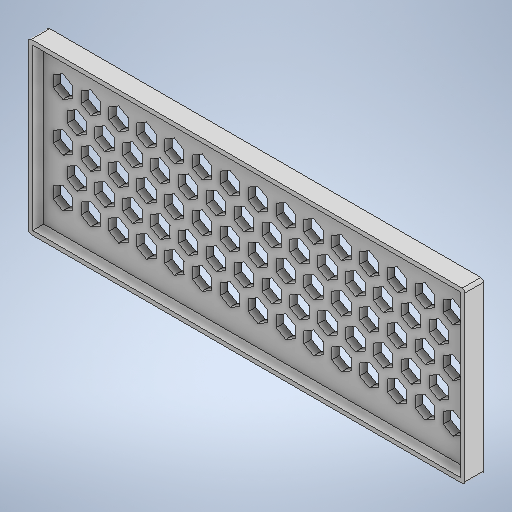
# Autodesk Inventor part: lm2596_box_lid_test
Saved by Autodesk Inventor 2025 (Build 290162000, 162)
## iProperties
Created: 2025-01-26
Part Number: lm2596_box_lid_test
Material: Všeobecné
Document SubType Name: Modeling
Designer: lukas
Density: 1 g/cm^3
Appearance: Výchozí
Author: lukas
## iProperties of the stored document lm2596_box_lid_3D tisk.ipt
Created: 2025-01-26
Part Number: lm2596_box_lid_3D tisk
Material: Všeobecné
Document SubType Name: Modeling
Designer: lukas
Density: 1 g/cm^3
Appearance: Výchozí
Author: lukas
Autodesk Inventor part; units mm, degrees
ref_plane "YZ Plane" through (0, 0, 0) normal (1, 0, 0) x (0, 1, 0)
ref_plane "XZ Plane" through (0, 0, 0) normal (0, 1, 0) x (-1, 0, 0)
ref_plane "XY Plane" through (0, 0, 0) normal (0, 0, 1) x (1, 0, 0)
sketch "Náčrt1" plane through (0, 0, 0) normal (0, 0, 1) x (1, 0, 0)
  line L0 (-117.5, 45.5) -> (117.5, 45.5)
  line L1 (117.5, 45.5) -> (117.5, -45.5)
  line L2 (117.5, -45.5) -> (-117.5, -45.5)
  line L3 (-117.5, -45.5) -> (-117.5, 45.5)
  line L4 (0, 63.7) -> (0, -63.7) projected
  line L5 (-164.5, 0) -> (164.5, 0) projected
  point P0 (0, 0)
  dimension "d0" = 235
  dimension "d1" = 91
  constraints: 8 end point, 2 parallel, 1 horizontal, 1 perpendicular, 2 other
  measures "d0" distance of L1.end L2.end
  measures "d1" distance of L0.end L1.end
extrude "Vysunutí1" add sketch "Náčrt1" along normal blind 4
sketch "Náčrt2" plane through (0, 0, 4) normal (0, 0, 1) x (1, 0, 0)
  line L0 (-117.5, 45.5) -> (-117.5, -45.5) projected
  line L1 (-117.5, -45.5) -> (117.5, -45.5) projected
  line L2 (117.5, -45.5) -> (117.5, 45.5) projected
  line L3 (117.5, 45.5) -> (-117.5, 45.5) projected
  line L4 (-164.5, 0) -> (164.5, 0) projected
  line L5 (0, -63.7) -> (0, 63.7) projected
  line L6 (-115.25, 43.25) -> (-115.25, -43.25)
  line L7 (-115.25, -43.25) -> (115.25, -43.25)
  line L8 (115.25, -43.25) -> (115.25, 43.25)
  line L9 (115.25, 43.25) -> (-115.25, 43.25)
  line L10 (-117.5, 45.5) -> (117.5, 45.5)
  line L11 (117.5, 45.5) -> (117.5, -45.5)
  line L12 (117.5, -45.5) -> (-117.5, -45.5)
  line L13 (-117.5, -45.5) -> (-117.5, 45.5)
  point P0 (0, 0)
  dimension "d5" = 2.25
  constraints: 16 end point, 2 parallel, 1 horizontal, 1 perpendicular, 3 other
  measures "d5" distance between parallel lines of L3 L9
extrude "Vysunutí2" add sketch "Náčrt2" along normal blind 6 contours L3 L5 L9 L6 L4 L0 | L4 L6 L7 L5 L1 L0 | L3 L2 L4 L8 L9 L5 | L5 L7 L8 L4 L2 L1
fillet "Zaoblení2" radius 1.5 4 edges at (117.5, -45.5, 5) (117.5, 45.5, 5) (-117.5, -45.5, 5) (-117.5, 45.5, 5)
sketch "Náčrt6" plane through (0, 0, 0) normal (0, 0, -1) x (-1, 0, 0)
  arc A0 (117.5, 44) -> (116, 45.5) centre (116, 44) ccw projected
  line L0 (-116, 45.5) -> (116, 45.5) projected
  arc A1 (-116, 45.5) -> (-117.5, 44) centre (-116, 44) ccw projected
  line L1 (-117.5, -44) -> (-117.5, 44) projected
  arc A2 (-117.5, -44) -> (-116, -45.5) centre (-116, -44) ccw projected
  line L2 (116, -45.5) -> (-116, -45.5) projected
  arc A3 (116, -45.5) -> (117.5, -44) centre (116, -44) ccw projected
  line L3 (117.5, 44) -> (117.5, -44) projected
  line L4 (0, -64.1349) -> (0, 64.1349) projected
  line L5 (-164.9349, 0) -> (164.9349, 0) projected
  line L6 (0, 6) -> (5.1962, 3)
  line L7 (5.1962, 3) -> (5.1962, -3)
  line L8 (5.1962, -3) -> (0, -6)
  line L9 (0, -6) -> (-5.1962, -3)
  line L10 (-5.1962, -3) -> (-5.1962, 3)
  line L11 (-5.1962, 3) -> (0, 6)
  line L12 (0, 0) -> (-2.5981, -4.5) construction
  line L13 (-7.5, -12.9904) -> (-10.0981, -17.4904) construction
  line L14 (-7.5, -18.9904) -> (-12.6962, -15.9904)
  line L15 (-12.6962, -15.9904) -> (-12.6962, -9.9904)
  line L16 (-2.3038, -9.9904) -> (-2.3038, -15.9904)
  line L17 (-12.6962, -9.9904) -> (-7.5, -6.9904)
  line L18 (-7.5, -6.9904) -> (-2.3038, -9.9904)
  line L19 (-2.3038, -15.9904) -> (-7.5, -18.9904)
  line L20 (-20.1962, 3) -> (-15, 6)
  line L21 (-15, 6) -> (-9.8038, 3)
  line L22 (-20.1962, -3) -> (-20.1962, 3)
  line L23 (-15, -6) -> (-20.1962, -3)
  line L24 (-9.8038, -3) -> (-15, -6)
  line L25 (-9.8038, 3) -> (-9.8038, -3)
  line L26 (9.8038, 3) -> (15, 6)
  line L27 (15, 6) -> (20.1962, 3)
  line L28 (9.8038, -3) -> (9.8038, 3)
  line L29 (15, -6) -> (9.8038, -3)
  line L30 (20.1962, -3) -> (15, -6)
  line L31 (20.1962, 3) -> (20.1962, -3)
  line L32 (-35.1962, 3) -> (-30, 6)
  line L33 (-30, 6) -> (-24.8038, 3)
  line L34 (-35.1962, -3) -> (-35.1962, 3)
  line L35 (-30, -6) -> (-35.1962, -3)
  line L36 (-24.8038, -3) -> (-30, -6)
  line L37 (-24.8038, 3) -> (-24.8038, -3)
  line L38 (24.8038, 3) -> (30, 6)
  line L39 (30, 6) -> (35.1962, 3)
  line L40 (24.8038, -3) -> (24.8038, 3)
  line L41 (30, -6) -> (24.8038, -3)
  line L42 (35.1962, -3) -> (30, -6)
  line L43 (35.1962, 3) -> (35.1962, -3)
  line L44 (-50.1962, 3) -> (-45, 6)
  line L45 (-45, 6) -> (-39.8038, 3)
  line L46 (-50.1962, -3) -> (-50.1962, 3)
  line L47 (-45, -6) -> (-50.1962, -3)
  line L48 (-39.8038, -3) -> (-45, -6)
  line L49 (-39.8038, 3) -> (-39.8038, -3)
  line L50 (39.8038, 3) -> (45, 6)
  line L51 (45, 6) -> (50.1962, 3)
  line L52 (39.8038, -3) -> (39.8038, 3)
  line L53 (45, -6) -> (39.8038, -3)
  line L54 (50.1962, -3) -> (45, -6)
  line L55 (50.1962, 3) -> (50.1962, -3)
  line L56 (-65.1962, 3) -> (-60, 6)
  line L57 (-60, 6) -> (-54.8038, 3)
  line L58 (-65.1962, -3) -> (-65.1962, 3)
  line L59 (-60, -6) -> (-65.1962, -3)
  line L60 (-54.8038, -3) -> (-60, -6)
  line L61 (-54.8038, 3) -> (-54.8038, -3)
  line L62 (54.8038, 3) -> (60, 6)
  line L63 (60, 6) -> (65.1962, 3)
  line L64 (54.8038, -3) -> (54.8038, 3)
  line L65 (60, -6) -> (54.8038, -3)
  line L66 (65.1962, -3) -> (60, -6)
  line L67 (65.1962, 3) -> (65.1962, -3)
  line L68 (-80.1962, 3) -> (-75, 6)
  line L69 (-75, 6) -> (-69.8038, 3)
  line L70 (-80.1962, -3) -> (-80.1962, 3)
  line L71 (-75, -6) -> (-80.1962, -3)
  line L72 (-69.8038, -3) -> (-75, -6)
  line L73 (-69.8038, 3) -> (-69.8038, -3)
  line L74 (69.8038, 3) -> (75, 6)
  line L75 (75, 6) -> (80.1962, 3)
  line L76 (69.8038, -3) -> (69.8038, 3)
  line L77 (75, -6) -> (69.8038, -3)
  line L78 (80.1962, -3) -> (75, -6)
  line L79 (80.1962, 3) -> (80.1962, -3)
  line L80 (-95.1962, 3) -> (-90, 6)
  line L81 (-90, 6) -> (-84.8038, 3)
  line L82 (-95.1962, -3) -> (-95.1962, 3)
  line L83 (-90, -6) -> (-95.1962, -3)
  line L84 (-84.8038, -3) -> (-90, -6)
  line L85 (-84.8038, 3) -> (-84.8038, -3)
  line L86 (84.8038, 3) -> (90, 6)
  line L87 (90, 6) -> (95.1962, 3)
  line L88 (84.8038, -3) -> (84.8038, 3)
  line L89 (90, -6) -> (84.8038, -3)
  line L90 (95.1962, -3) -> (90, -6)
  line L91 (95.1962, 3) -> (95.1962, -3)
  line L92 (-110.1962, 3) -> (-105, 6)
  line L93 (-105, 6) -> (-99.8038, 3)
  line L94 (-110.1962, -3) -> (-110.1962, 3)
  line L95 (-105, -6) -> (-110.1962, -3)
  line L96 (-99.8038, -3) -> (-105, -6)
  line L97 (-99.8038, 3) -> (-99.8038, -3)
  line L98 (99.8038, 3) -> (105, 6)
  line L99 (105, 6) -> (110.1962, 3)
  line L100 (99.8038, -3) -> (99.8038, 3)
  line L101 (105, -6) -> (99.8038, -3)
  line L102 (110.1962, -3) -> (105, -6)
  line L103 (110.1962, 3) -> (110.1962, -3)
  line L104 (7.5, -12.9904) -> (4.9019, -17.4904) construction
  line L105 (2.3038, -9.9904) -> (7.5, -6.9904)
  line L106 (2.3038, -15.9904) -> (2.3038, -9.9904)
  line L107 (7.5, -18.9904) -> (2.3038, -15.9904)
  line L108 (12.6962, -15.9904) -> (7.5, -18.9904)
  line L109 (7.5, -6.9904) -> (12.6962, -9.9904)
  line L110 (12.6962, -9.9904) -> (12.6962, -15.9904)
  line L111 (22.5, -12.9904) -> (19.9019, -17.4904) construction
  line L112 (17.3038, -9.9904) -> (22.5, -6.9904)
  line L113 (17.3038, -15.9904) -> (17.3038, -9.9904)
  line L114 (22.5, -18.9904) -> (17.3038, -15.9904)
  line L115 (27.6962, -15.9904) -> (22.5, -18.9904)
  line L116 (22.5, -6.9904) -> (27.6962, -9.9904)
  line L117 (27.6962, -9.9904) -> (27.6962, -15.9904)
  line L118 (37.5, -12.9904) -> (34.9019, -17.4904) construction
  line L119 (32.3038, -9.9904) -> (37.5, -6.9904)
  line L120 (32.3038, -15.9904) -> (32.3038, -9.9904)
  line L121 (37.5, -18.9904) -> (32.3038, -15.9904)
  line L122 (42.6962, -15.9904) -> (37.5, -18.9904)
  line L123 (37.5, -6.9904) -> (42.6962, -9.9904)
  line L124 (42.6962, -9.9904) -> (42.6962, -15.9904)
  line L125 (52.5, -12.9904) -> (49.9019, -17.4904) construction
  line L126 (47.3038, -9.9904) -> (52.5, -6.9904)
  line L127 (47.3038, -15.9904) -> (47.3038, -9.9904)
  line L128 (52.5, -18.9904) -> (47.3038, -15.9904)
  line L129 (57.6962, -15.9904) -> (52.5, -18.9904)
  line L130 (52.5, -6.9904) -> (57.6962, -9.9904)
  line L131 (57.6962, -9.9904) -> (57.6962, -15.9904)
  line L132 (67.5, -12.9904) -> (64.9019, -17.4904) construction
  line L133 (62.3038, -9.9904) -> (67.5, -6.9904)
  line L134 (62.3038, -15.9904) -> (62.3038, -9.9904)
  line L135 (67.5, -18.9904) -> (62.3038, -15.9904)
  line L136 (72.6962, -15.9904) -> (67.5, -18.9904)
  line L137 (67.5, -6.9904) -> (72.6962, -9.9904)
  line L138 (72.6962, -9.9904) -> (72.6962, -15.9904)
  line L139 (82.5, -12.9904) -> (79.9019, -17.4904) construction
  line L140 (77.3038, -9.9904) -> (82.5, -6.9904)
  line L141 (77.3038, -15.9904) -> (77.3038, -9.9904)
  line L142 (82.5, -18.9904) -> (77.3038, -15.9904)
  line L143 (87.6962, -15.9904) -> (82.5, -18.9904)
  line L144 (82.5, -6.9904) -> (87.6962, -9.9904)
  line L145 (87.6962, -9.9904) -> (87.6962, -15.9904)
  line L146 (97.5, -12.9904) -> (94.9019, -17.4904) construction
  line L147 (92.3038, -9.9904) -> (97.5, -6.9904)
  line L148 (92.3038, -15.9904) -> (92.3038, -9.9904)
  line L149 (97.5, -18.9904) -> (92.3038, -15.9904)
  line L150 (102.6962, -15.9904) -> (97.5, -18.9904)
  line L151 (97.5, -6.9904) -> (102.6962, -9.9904)
  line L152 (102.6962, -9.9904) -> (102.6962, -15.9904)
  line L153 (-27.6962, -9.9904) -> (-22.5, -6.9904)
  line L154 (-22.5, -6.9904) -> (-17.3038, -9.9904)
  line L155 (-27.6962, -15.9904) -> (-27.6962, -9.9904)
  line L156 (-22.5, -12.9904) -> (-25.0981, -17.4904) construction
  line L157 (-22.5, -18.9904) -> (-27.6962, -15.9904)
  line L158 (-17.3038, -15.9904) -> (-22.5, -18.9904)
  line L159 (-17.3038, -9.9904) -> (-17.3038, -15.9904)
  line L160 (-42.6962, -9.9904) -> (-37.5, -6.9904)
  line L161 (-37.5, -6.9904) -> (-32.3038, -9.9904)
  line L162 (-42.6962, -15.9904) -> (-42.6962, -9.9904)
  line L163 (-37.5, -12.9904) -> (-40.0981, -17.4904) construction
  line L164 (-37.5, -18.9904) -> (-42.6962, -15.9904)
  line L165 (-32.3038, -15.9904) -> (-37.5, -18.9904)
  line L166 (-32.3038, -9.9904) -> (-32.3038, -15.9904)
  line L167 (-57.6962, -9.9904) -> (-52.5, -6.9904)
  line L168 (-52.5, -6.9904) -> (-47.3038, -9.9904)
  line L169 (-57.6962, -15.9904) -> (-57.6962, -9.9904)
  line L170 (-52.5, -12.9904) -> (-55.0981, -17.4904) construction
  line L171 (-52.5, -18.9904) -> (-57.6962, -15.9904)
  line L172 (-47.3038, -15.9904) -> (-52.5, -18.9904)
  line L173 (-47.3038, -9.9904) -> (-47.3038, -15.9904)
  line L174 (-72.6962, -9.9904) -> (-67.5, -6.9904)
  line L175 (-67.5, -6.9904) -> (-62.3038, -9.9904)
  line L176 (-72.6962, -15.9904) -> (-72.6962, -9.9904)
  line L177 (-67.5, -12.9904) -> (-70.0981, -17.4904) construction
  line L178 (-67.5, -18.9904) -> (-72.6962, -15.9904)
  line L179 (-62.3038, -15.9904) -> (-67.5, -18.9904)
  line L180 (-62.3038, -9.9904) -> (-62.3038, -15.9904)
  line L181 (-87.6962, -9.9904) -> (-82.5, -6.9904)
  line L182 (-82.5, -6.9904) -> (-77.3038, -9.9904)
  line L183 (-87.6962, -15.9904) -> (-87.6962, -9.9904)
  line L184 (-82.5, -12.9904) -> (-85.0981, -17.4904) construction
  line L185 (-82.5, -18.9904) -> (-87.6962, -15.9904)
  line L186 (-77.3038, -15.9904) -> (-82.5, -18.9904)
  line L187 (-77.3038, -9.9904) -> (-77.3038, -15.9904)
  line L188 (-102.6962, -9.9904) -> (-97.5, -6.9904)
  line L189 (-97.5, -6.9904) -> (-92.3038, -9.9904)
  line L190 (-102.6962, -15.9904) -> (-102.6962, -9.9904)
  line L191 (-97.5, -12.9904) -> (-100.0981, -17.4904) construction
  line L192 (-97.5, -18.9904) -> (-102.6962, -15.9904)
  line L193 (-92.3038, -15.9904) -> (-97.5, -18.9904)
  line L194 (-92.3038, -9.9904) -> (-92.3038, -15.9904)
  line L195 (-12.6962, 15.9896) -> (-7.5, 18.9896)
  line L196 (-7.5, 18.9896) -> (-2.3038, 15.9896)
  line L197 (-2.3038, 15.9896) -> (-2.3038, 9.9896)
  line L198 (-2.3038, 9.9896) -> (-7.5, 6.9896)
  line L199 (-7.5, 12.9896) -> (-10.0981, 8.4896) construction
  line L200 (-7.5, 6.9896) -> (-12.6962, 9.9896)
  line L201 (-12.6962, 9.9896) -> (-12.6962, 15.9896)
  line L202 (2.3038, 9.9896) -> (2.3038, 15.9896)
  line L203 (7.5, 6.9896) -> (2.3038, 9.9896)
  line L204 (2.3038, 15.9896) -> (7.5, 18.9896)
  line L205 (7.5, 12.9896) -> (4.9019, 8.4896) construction
  line L206 (12.6962, 9.9896) -> (7.5, 6.9896)
  line L207 (12.6962, 15.9896) -> (12.6962, 9.9896)
  line L208 (7.5, 18.9896) -> (12.6962, 15.9896)
  line L209 (32.3038, 15.9896) -> (37.5, 18.9896)
  line L210 (37.5, 18.9896) -> (42.6962, 15.9896)
  line L211 (32.3038, 9.9896) -> (32.3038, 15.9896)
  line L212 (42.6962, 15.9896) -> (42.6962, 9.9896)
  line L213 (37.5, 12.9896) -> (34.9019, 8.4896) construction
  line L214 (37.5, 6.9896) -> (32.3038, 9.9896)
  line L215 (42.6962, 9.9896) -> (37.5, 6.9896)
  line L216 (-42.6962, 15.9896) -> (-37.5, 18.9896)
  line L217 (-37.5, 18.9896) -> (-32.3038, 15.9896)
  line L218 (-32.3038, 15.9896) -> (-32.3038, 9.9896)
  line L219 (-32.3038, 9.9896) -> (-37.5, 6.9896)
  line L220 (-37.5, 12.9896) -> (-40.0981, 8.4896) construction
  line L221 (-42.6962, 9.9896) -> (-42.6962, 15.9896)
  line L222 (-37.5, 6.9896) -> (-42.6962, 9.9896)
  line L223 (62.3038, 15.9896) -> (67.5, 18.9896)
  line L224 (62.3038, 9.9896) -> (62.3038, 15.9896)
  line L225 (67.5, 18.9896) -> (72.6962, 15.9896)
  line L226 (67.5, 6.9896) -> (62.3038, 9.9896)
  line L227 (72.6962, 15.9896) -> (72.6962, 9.9896)
  line L228 (72.6962, 9.9896) -> (67.5, 6.9896)
  line L229 (67.5, 12.9896) -> (64.9019, 8.4896) construction
  line L230 (-67.5, 18.9896) -> (-62.3038, 15.9896)
  line L231 (-57.6962, 15.9896) -> (-52.5, 18.9896)
  line L232 (-62.3038, 15.9896) -> (-62.3038, 9.9896)
  line L233 (-62.3038, 9.9896) -> (-67.5, 6.9896)
  line L234 (-52.5, 18.9896) -> (-47.3038, 15.9896)
  line L235 (-57.6962, 9.9896) -> (-57.6962, 15.9896)
  line L236 (-52.5, 12.9896) -> (-55.0981, 8.4896) construction
  line L237 (-47.3038, 15.9896) -> (-47.3038, 9.9896)
  line L238 (-47.3038, 9.9896) -> (-52.5, 6.9896)
  line L239 (-52.5, 6.9896) -> (-57.6962, 9.9896)
  line L240 (-82.5, 12.9896) -> (-85.0981, 8.4896) construction
  line L241 (-82.5, 6.9896) -> (-87.6962, 9.9896)
  line L242 (-87.6962, 15.9896) -> (-82.5, 18.9896)
  line L243 (-87.6962, 9.9896) -> (-87.6962, 15.9896)
  line L244 (92.3038, 15.9896) -> (97.5, 18.9896)
  line L245 (87.6962, 15.9896) -> (87.6962, 9.9896)
  line L246 (92.3038, 9.9896) -> (92.3038, 15.9896)
  line L247 (97.5, 18.9896) -> (102.6962, 15.9896)
  line L248 (97.5, 12.9896) -> (94.9019, 8.4896) construction
  line L249 (97.5, 6.9896) -> (92.3038, 9.9896)
  line L250 (102.6962, 15.9896) -> (102.6962, 9.9896)
  line L251 (102.6962, 9.9896) -> (97.5, 6.9896)
  line L252 (77.3038, 9.9896) -> (77.3038, 15.9896)
  line L253 (82.5, 6.9896) -> (77.3038, 9.9896)
  line L254 (82.5, 12.9896) -> (79.9019, 8.4896) construction
  line L255 (77.3038, 15.9896) -> (82.5, 18.9896)
  line L256 (82.5, 18.9896) -> (87.6962, 15.9896)
  line L257 (87.6962, 9.9896) -> (82.5, 6.9896)
  line L258 (-102.6962, 15.9896) -> (-97.5, 18.9896)
  line L259 (-97.5, 18.9896) -> (-92.3038, 15.9896)
  line L260 (-102.6962, 9.9896) -> (-102.6962, 15.9896)
  line L261 (-97.5, 12.9896) -> (-100.0981, 8.4896) construction
  line L262 (-97.5, 6.9896) -> (-102.6962, 9.9896)
  line L263 (-92.3038, 15.9896) -> (-92.3038, 9.9896)
  line L264 (-92.3038, 9.9896) -> (-97.5, 6.9896)
  line L265 (47.3038, 9.9896) -> (47.3038, 15.9896)
  line L266 (47.3038, 15.9896) -> (52.5, 18.9896)
  line L267 (52.5, 6.9896) -> (47.3038, 9.9896)
  line L268 (52.5, 12.9896) -> (49.9019, 8.4896) construction
  line L269 (52.5, 18.9896) -> (57.6962, 15.9896)
  line L270 (57.6962, 15.9896) -> (57.6962, 9.9896)
  line L271 (57.6962, 9.9896) -> (52.5, 6.9896)
  line L272 (-27.6962, 9.9896) -> (-27.6962, 15.9896)
  line L273 (-27.6962, 15.9896) -> (-22.5, 18.9896)
  line L274 (-22.5, 18.9896) -> (-17.3038, 15.9896)
  line L275 (-22.5, 12.9896) -> (-25.0981, 8.4896) construction
  line L276 (-22.5, 6.9896) -> (-27.6962, 9.9896)
  line L277 (-17.3038, 15.9896) -> (-17.3038, 9.9896)
  line L278 (-17.3038, 9.9896) -> (-22.5, 6.9896)
  line L279 (-77.3038, 9.9896) -> (-82.5, 6.9896)
  line L280 (-82.5, 18.9896) -> (-77.3038, 15.9896)
  line L281 (-77.3038, 15.9896) -> (-77.3038, 9.9896)
  line L282 (-72.6962, 9.9896) -> (-72.6962, 15.9896)
  line L283 (-72.6962, 15.9896) -> (-67.5, 18.9896)
  line L284 (-67.5, 12.9896) -> (-70.0981, 8.4896) construction
  line L285 (-67.5, 6.9896) -> (-72.6962, 9.9896)
  line L286 (17.3038, 9.9896) -> (17.3038, 15.9896)
  line L287 (22.5, 6.9896) -> (17.3038, 9.9896)
  line L288 (17.3038, 15.9896) -> (22.5, 18.9896)
  line L289 (22.5, 12.9896) -> (19.9019, 8.4896) construction
  line L290 (27.6962, 15.9896) -> (27.6962, 9.9896)
  line L291 (22.5, 18.9896) -> (27.6962, 15.9896)
  line L292 (27.6962, 9.9896) -> (22.5, 6.9896)
  line L293 (84.8038, 28.98) -> (90, 31.98)
  line L294 (75, 31.98) -> (80.1962, 28.98)
  line L295 (-50.1962, 22.98) -> (-50.1962, 28.98)
  line L296 (-65.1962, 28.98) -> (-60, 31.98)
  line L297 (-60, 31.98) -> (-54.8038, 28.98)
  line L298 (-60, 19.98) -> (-65.1962, 22.98)
  line L299 (-54.8038, 22.98) -> (-60, 19.98)
  line L300 (-54.8038, 28.98) -> (-54.8038, 22.98)
  line L301 (-69.8038, 28.98) -> (-69.8038, 22.98)
  line L302 (-75, 31.98) -> (-69.8038, 28.98)
  line L303 (-45, 19.98) -> (-50.1962, 22.98)
  line L304 (-39.8038, 22.98) -> (-45, 19.98)
  line L305 (-35.1962, 28.98) -> (-30, 31.98)
  line L306 (-30, 31.98) -> (-24.8038, 28.98)
  line L307 (-35.1962, 22.98) -> (-35.1962, 28.98)
  line L308 (-39.8038, 28.98) -> (-39.8038, 22.98)
  line L309 (-24.8038, 28.98) -> (-24.8038, 22.98)
  line L310 (-30, 19.98) -> (-35.1962, 22.98)
  line L311 (-24.8038, 22.98) -> (-30, 19.98)
  line L312 (-5.1962, 22.98) -> (-5.1962, 28.98)
  line L313 (-20.1962, 28.98) -> (-15, 31.98)
  line L314 (-15, 31.98) -> (-9.8038, 28.98)
  line L315 (-20.1962, 22.98) -> (-20.1962, 28.98)
  line L316 (-15, 19.98) -> (-20.1962, 22.98)
  line L317 (-9.8038, 28.98) -> (-9.8038, 22.98)
  line L318 (-9.8038, 22.98) -> (-15, 19.98)
  line L319 (-5.1962, 28.98) -> (0, 31.98)
  line L320 (0, 25.98) -> (-2.5981, 21.48) construction
  line L321 (5.1962, 28.98) -> (5.1962, 22.98)
  line L322 (0, 31.98) -> (5.1962, 28.98)
  line L323 (5.1962, 22.98) -> (0, 19.98)
  line L324 (0, 19.98) -> (-5.1962, 22.98)
  line L325 (15, 19.98) -> (9.8038, 22.98)
  line L326 (9.8038, 28.98) -> (15, 31.98)
  line L327 (15, 31.98) -> (20.1962, 28.98)
  line L328 (9.8038, 22.98) -> (9.8038, 28.98)
  line L329 (20.1962, 22.98) -> (15, 19.98)
  line L330 (20.1962, 28.98) -> (20.1962, 22.98)
  line L331 (24.8038, 28.98) -> (30, 31.98)
  line L332 (24.8038, 22.98) -> (24.8038, 28.98)
  line L333 (30, 19.98) -> (24.8038, 22.98)
  line L334 (30, 31.98) -> (35.1962, 28.98)
  line L335 (35.1962, 22.98) -> (30, 19.98)
  line L336 (45, 19.98) -> (39.8038, 22.98)
  line L337 (50.1962, 22.98) -> (45, 19.98)
  line L338 (50.1962, 28.98) -> (50.1962, 22.98)
  line L339 (45, 31.98) -> (50.1962, 28.98)
  line L340 (39.8038, 22.98) -> (39.8038, 28.98)
  line L341 (35.1962, 28.98) -> (35.1962, 22.98)
  line L342 (39.8038, 28.98) -> (45, 31.98)
  line L343 (54.8038, 22.98) -> (54.8038, 28.98)
  line L344 (60, 19.98) -> (54.8038, 22.98)
  line L345 (54.8038, 28.98) -> (60, 31.98)
  line L346 (60, 31.98) -> (65.1962, 28.98)
  line L347 (65.1962, 22.98) -> (60, 19.98)
  line L348 (75, 19.98) -> (69.8038, 22.98)
  line L349 (80.1962, 22.98) -> (75, 19.98)
  line L350 (69.8038, 22.98) -> (69.8038, 28.98)
  line L351 (65.1962, 28.98) -> (65.1962, 22.98)
  line L352 (69.8038, 28.98) -> (75, 31.98)
  line L353 (80.1962, 28.98) -> (80.1962, 22.98)
  line L354 (84.8038, 22.98) -> (84.8038, 28.98)
  line L355 (90, 19.98) -> (84.8038, 22.98)
  line L356 (105, 19.98) -> (99.8038, 22.98)
  line L357 (95.1962, 22.98) -> (90, 19.98)
  line L358 (95.1962, 28.98) -> (95.1962, 22.98)
  line L359 (90, 31.98) -> (95.1962, 28.98)
  line L360 (110.1962, 22.98) -> (105, 19.98)
  line L361 (99.8038, 22.98) -> (99.8038, 28.98)
  line L362 (110.1962, 28.98) -> (110.1962, 22.98)
  line L363 (99.8038, 28.98) -> (105, 31.98)
  line L364 (105, 31.98) -> (110.1962, 28.98)
  line L365 (-45, 31.98) -> (-39.8038, 28.98)
  line L366 (-50.1962, 28.98) -> (-45, 31.98)
  line L367 (-95.1962, 28.98) -> (-90, 31.98)
  line L368 (-90, 31.98) -> (-84.8038, 28.98)
  line L369 (-95.1962, 22.98) -> (-95.1962, 28.98)
  line L370 (-90, 19.98) -> (-95.1962, 22.98)
  line L371 (-105, 31.98) -> (-99.8038, 28.98)
  line L372 (-84.8038, 28.98) -> (-84.8038, 22.98)
  line L373 (-84.8038, 22.98) -> (-90, 19.98)
  line L374 (-110.1962, 28.98) -> (-105, 31.98)
  line L375 (-99.8038, 28.98) -> (-99.8038, 22.98)
  line L376 (-99.8038, 22.98) -> (-105, 19.98)
  line L377 (-110.1962, 22.98) -> (-110.1962, 28.98)
  line L378 (-105, 19.98) -> (-110.1962, 22.98)
  line L379 (-75, 19.98) -> (-80.1962, 22.98)
  line L380 (-80.1962, 22.98) -> (-80.1962, 28.98)
  line L381 (-80.1962, 28.98) -> (-75, 31.98)
  line L382 (-65.1962, 22.98) -> (-65.1962, 28.98)
  line L383 (-69.8038, 22.98) -> (-75, 19.98)
  line L384 (84.8038, -22.98) -> (90, -19.98)
  line L385 (75, -19.98) -> (80.1962, -22.98)
  line L386 (-50.1962, -28.98) -> (-50.1962, -22.98)
  line L387 (-65.1962, -22.98) -> (-60, -19.98)
  line L388 (-60, -19.98) -> (-54.8038, -22.98)
  line L389 (-60, -31.98) -> (-65.1962, -28.98)
  line L390 (-54.8038, -28.98) -> (-60, -31.98)
  line L391 (-54.8038, -22.98) -> (-54.8038, -28.98)
  line L392 (-69.8038, -22.98) -> (-69.8038, -28.98)
  line L393 (-75, -19.98) -> (-69.8038, -22.98)
  line L394 (-45, -31.98) -> (-50.1962, -28.98)
  line L395 (-39.8038, -28.98) -> (-45, -31.98)
  line L396 (-35.1962, -22.98) -> (-30, -19.98)
  line L397 (-30, -19.98) -> (-24.8038, -22.98)
  line L398 (-35.1962, -28.98) -> (-35.1962, -22.98)
  line L399 (-39.8038, -22.98) -> (-39.8038, -28.98)
  line L400 (-24.8038, -22.98) -> (-24.8038, -28.98)
  line L401 (-30, -31.98) -> (-35.1962, -28.98)
  line L402 (-24.8038, -28.98) -> (-30, -31.98)
  line L403 (-5.1962, -28.98) -> (-5.1962, -22.98)
  line L404 (-20.1962, -22.98) -> (-15, -19.98)
  line L405 (-15, -19.98) -> (-9.8038, -22.98)
  line L406 (-20.1962, -28.98) -> (-20.1962, -22.98)
  line L407 (-15, -31.98) -> (-20.1962, -28.98)
  line L408 (-9.8038, -22.98) -> (-9.8038, -28.98)
  line L409 (-9.8038, -28.98) -> (-15, -31.98)
  line L410 (-5.1962, -22.98) -> (0, -19.98)
  line L411 (0, -25.98) -> (-2.5981, -30.48) construction
  line L412 (5.1962, -22.98) -> (5.1962, -28.98)
  line L413 (0, -19.98) -> (5.1962, -22.98)
  line L414 (5.1962, -28.98) -> (0, -31.98)
  line L415 (0, -31.98) -> (-5.1962, -28.98)
  line L416 (15, -31.98) -> (9.8038, -28.98)
  line L417 (9.8038, -22.98) -> (15, -19.98)
  line L418 (15, -19.98) -> (20.1962, -22.98)
  line L419 (9.8038, -28.98) -> (9.8038, -22.98)
  line L420 (20.1962, -28.98) -> (15, -31.98)
  line L421 (20.1962, -22.98) -> (20.1962, -28.98)
  line L422 (24.8038, -22.98) -> (30, -19.98)
  line L423 (24.8038, -28.98) -> (24.8038, -22.98)
  line L424 (30, -31.98) -> (24.8038, -28.98)
  line L425 (30, -19.98) -> (35.1962, -22.98)
  line L426 (35.1962, -28.98) -> (30, -31.98)
  line L427 (45, -31.98) -> (39.8038, -28.98)
  line L428 (50.1962, -28.98) -> (45, -31.98)
  line L429 (50.1962, -22.98) -> (50.1962, -28.98)
  line L430 (45, -19.98) -> (50.1962, -22.98)
  line L431 (39.8038, -28.98) -> (39.8038, -22.98)
  line L432 (35.1962, -22.98) -> (35.1962, -28.98)
  line L433 (39.8038, -22.98) -> (45, -19.98)
  line L434 (54.8038, -28.98) -> (54.8038, -22.98)
  line L435 (60, -31.98) -> (54.8038, -28.98)
  line L436 (54.8038, -22.98) -> (60, -19.98)
  line L437 (60, -19.98) -> (65.1962, -22.98)
  line L438 (65.1962, -28.98) -> (60, -31.98)
  line L439 (75, -31.98) -> (69.8038, -28.98)
  line L440 (80.1962, -28.98) -> (75, -31.98)
  line L441 (69.8038, -28.98) -> (69.8038, -22.98)
  line L442 (65.1962, -22.98) -> (65.1962, -28.98)
  line L443 (69.8038, -22.98) -> (75, -19.98)
  line L444 (80.1962, -22.98) -> (80.1962, -28.98)
  line L445 (84.8038, -28.98) -> (84.8038, -22.98)
  line L446 (90, -31.98) -> (84.8038, -28.98)
  line L447 (105, -31.98) -> (99.8038, -28.98)
  line L448 (95.1962, -28.98) -> (90, -31.98)
  line L449 (95.1962, -22.98) -> (95.1962, -28.98)
  line L450 (90, -19.98) -> (95.1962, -22.98)
  line L451 (110.1962, -28.98) -> (105, -31.98)
  line L452 (99.8038, -28.98) -> (99.8038, -22.98)
  line L453 (110.1962, -22.98) -> (110.1962, -28.98)
  line L454 (99.8038, -22.98) -> (105, -19.98)
  line L455 (105, -19.98) -> (110.1962, -22.98)
  line L456 (-45, -19.98) -> (-39.8038, -22.98)
  line L457 (-50.1962, -22.98) -> (-45, -19.98)
  line L458 (-95.1962, -22.98) -> (-90, -19.98)
  line L459 (-90, -19.98) -> (-84.8038, -22.98)
  line L460 (-95.1962, -28.98) -> (-95.1962, -22.98)
  line L461 (-90, -31.98) -> (-95.1962, -28.98)
  line L462 (-105, -19.98) -> (-99.8038, -22.98)
  line L463 (-84.8038, -22.98) -> (-84.8038, -28.98)
  line L464 (-84.8038, -28.98) -> (-90, -31.98)
  line L465 (-110.1962, -22.98) -> (-105, -19.98)
  line L466 (-99.8038, -22.98) -> (-99.8038, -28.98)
  line L467 (-99.8038, -28.98) -> (-105, -31.98)
  line L468 (-110.1962, -28.98) -> (-110.1962, -22.98)
  line L469 (-105, -31.98) -> (-110.1962, -28.98)
  line L470 (-75, -31.98) -> (-80.1962, -28.98)
  line L471 (-80.1962, -28.98) -> (-80.1962, -22.98)
  line L472 (-80.1962, -22.98) -> (-75, -19.98)
  line L473 (-65.1962, -28.98) -> (-65.1962, -22.98)
  line L474 (-69.8038, -28.98) -> (-75, -31.98)
  point P0 (-15, 0)
  point P1 (-17.5981, -4.5)
  point P2 (15, 0)
  point P3 (12.4019, -4.5)
  point P4 (-30, 0)
  point P5 (-32.5981, -4.5)
  point P6 (30, 0)
  point P7 (27.4019, -4.5)
  point P8 (-45, 0)
  point P9 (-47.5981, -4.5)
  point P10 (45, 0)
  point P11 (42.4019, -4.5)
  point P12 (-60, 0)
  point P13 (-62.5981, -4.5)
  point P14 (60, 0)
  point P15 (57.4019, -4.5)
  point P16 (-75, 0)
  point P17 (-77.5981, -4.5)
  point P18 (75, 0)
  point P19 (72.4019, -4.5)
  point P20 (-90, 0)
  point P21 (-92.5981, -4.5)
  point P22 (90, 0)
  point P23 (87.4019, -4.5)
  point P24 (-105, 0)
  point P25 (-107.5981, -4.5)
  point P26 (105, 0)
  point P27 (102.4019, -4.5)
  point P28 (-60, 25.98)
  point P29 (-62.5981, 21.48)
  point P30 (-47.5981, 21.48)
  point P31 (-32.5981, 21.48)
  point P32 (-15, 25.98)
  point P33 (-17.5981, 21.48)
  point P34 (12.4019, 21.48)
  point P35 (15, 25.98)
  point P36 (30, 25.98)
  point P37 (27.4019, 21.48)
  point P38 (42.4019, 21.48)
  point P39 (45, 25.98)
  point P40 (60, 25.98)
  point P41 (57.4019, 21.48)
  point P42 (72.4019, 21.48)
  point P43 (75, 25.98)
  point P44 (90, 25.98)
  point P45 (87.4019, 21.48)
  point P46 (102.4019, 21.48)
  point P47 (105, 25.98)
  point P48 (-30, 25.98)
  point P49 (-45, 25.98)
  point P50 (-90, 25.98)
  point P51 (-92.5981, 21.48)
  point P52 (-105, 25.98)
  point P53 (-107.5981, 21.48)
  point P54 (-77.5981, 21.48)
  point P55 (-75, 25.98)
  point P56 (-60, -25.98)
  point P57 (-62.5981, -30.48)
  point P58 (-47.5981, -30.48)
  point P59 (-32.5981, -30.48)
  point P60 (-15, -25.98)
  point P61 (-17.5981, -30.48)
  point P62 (12.4019, -30.48)
  point P63 (15, -25.98)
  point P64 (30, -25.98)
  point P65 (27.4019, -30.48)
  point P66 (42.4019, -30.48)
  point P67 (45, -25.98)
  point P68 (60, -25.98)
  point P69 (57.4019, -30.48)
  point P70 (72.4019, -30.48)
  point P71 (75, -25.98)
  point P72 (90, -25.98)
  point P73 (87.4019, -30.48)
  point P74 (102.4019, -30.48)
  point P75 (105, -25.98)
  point P76 (-30, -25.98)
  point P77 (-45, -25.98)
  point P78 (-90, -25.98)
  point P79 (-92.5981, -30.48)
  point P80 (-105, -25.98)
  point P81 (-107.5981, -30.48)
  point P82 (-77.5981, -30.48)
  point P83 (-75, -25.98)
  dimension "d62" = 6
  dimension "d65" = 15
  dimension "d72" = 15
  dimension "d79" = 15
  dimension "d86" = 15
  dimension "d93" = 25.98
  dimension "d100" = 25.98
  constraints: 938 end point, 3 horizontal, 2 vertical, 1 coincident, 1 collinear, 1 midpoint, 1 point on line, 1051 other
  measures "d62" distance of L6.end L7.end
  measures "d65" distance of L12.end L13.end
  measures "d72" distance of L12.start point (-15, 0)
  measures "d79" distance of L14.start L107.start
  measures "d86" distance of L17.end L153.end
  measures "d93" distance of L15.end L195.start
  measures "d100" distance of L86.start L293.start
extrude "Vysunutí6" cut sketch "Náčrt6" against normal blind 10 contours L103 L102 L101 L100 L5 | L5 L100 L98 L99 L103 | L322 L321 L323 L4 | L4 L324 L312 L319 | L91 L90 L89 L88 L5 | L5 L88 L86 L87 L91 | L6 L7 L5 L4 | L4 L5 L10 L11 | L415 L403 L410 L4 | L4 L413 L412 L414 | L94 L92 L93 L97 L5 | L5 L97 L96 L95 L94 | L5 L7 L8 L4 | L4 L9 L10 L5 | L79 L78 L77 L76 L5 | L5 L76 L74 L75 L79 | L82 L80 L81 L85 L5 | L5 L85 L84 L83 L82 | L25 L24 L23 L22 L5 | L5 L22 L20 L21 L25 | L28 L26 L27 L31 L5 | L5 L31 L30 L29 L28 | L67 L66 L65 L64 L5 | L5 L64 L62 L63 L67 | L70 L68 L69 L73 L5 | L5 L73 L72 L71 L70 | L37 L36 L35 L34 L5 | L5 L34 L32 L33 L37 | L40 L38 L39 L43 L5 | L5 L43 L42 L41 L40 | L55 L54 L53 L52 L5 | L5 L52 L50 L51 L55 | L58 L56 L57 L61 L5 | L5 L61 L60 L59 L58 | L49 L48 L47 L46 L5 | L5 L46 L44 L45 L49 | L14 L15 L17 L18 L16 L19 | L105 L109 L110 L108 L107 L106 | L112 L116 L117 L115 L114 L113 | L119 L123 L124 L122 L121 L120 | L126 L130 L131 L129 L128 L127 | L133 L137 L138 L136 L135 L134 | L140 L144 L145 L143 L142 L141 | L147 L151 L152 L150 L149 L148 | L153 L154 L159 L158 L157 L155 | L160 L161 L166 L165 L164 L162 | L167 L168 L173 L172 L171 L169 | L174 L175 L180 L179 L178 L176 | L181 L182 L187 L186 L185 L183 | L188 L189 L194 L193 L192 L190 | L195 L196 L197 L198 L200 L201 | L202 L204 L208 L207 L206 L203 | L209 L210 L212 L215 L214 L211 | L216 L217 L218 L219 L222 L221 | L223 L225 L227 L228 L226 L224 | L230 L232 L233 L285 L282 L283 | L231 L234 L237 L238 L239 L235 | L241 L243 L242 L280 L281 L279 | L244 L247 L250 L251 L249 L246 | L245 L257 L253 L252 L255 L256 | L258 L259 L263 L264 L262 L260 | L265 L266 L269 L270 L271 L267 | L272 L273 L274 L277 L278 L276 | L286 L288 L291 L290 L292 L287 | L293 L359 L358 L357 L355 L354 | L294 L353 L349 L348 L350 L352 | L295 L366 L365 L308 L304 L303 | L296 L297 L300 L299 L298 L382 | L301 L383 L379 L380 L381 L302 | L305 L306 L309 L311 L310 L307 | L313 L314 L317 L318 L316 L315 | L325 L328 L326 L327 L330 L329 | L331 L334 L341 L335 L333 L332 | L336 L340 L342 L339 L338 L337 | L343 L345 L346 L351 L347 L344 | L356 L361 L363 L364 L362 L360 | L367 L368 L372 L373 L370 L369 | L371 L375 L376 L378 L377 L374 | L384 L450 L449 L448 L446 L445 | L385 L444 L440 L439 L441 L443 | L386 L457 L456 L399 L395 L394 | L387 L388 L391 L390 L389 L473 | L392 L474 L470 L471 L472 L393 | L396 L397 L400 L402 L401 L398 | L404 L405 L408 L409 L407 L406 | L416 L419 L417 L418 L421 L420 | L422 L425 L432 L426 L424 L423 | L427 L431 L433 L430 L429 L428 | L434 L436 L437 L442 L438 L435 | L447 L452 L454 L455 L453 L451 | L458 L459 L463 L464 L461 L460 | L462 L466 L467 L469 L468 L465
